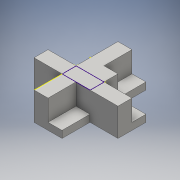
# Autodesk Inventor part: fourwayVer3
Saved by Autodesk Inventor 2016 (Build 200138000, 138)
## iProperties
Created: 2015-11-25
Part Number: fourwayVer3
Material: Generic
Document SubType Name: Modeling
Designer: hesaon
Density: 1 g/cm^3
Appearance: Default
Author: hesaon
Autodesk Inventor part; units mm, degrees
ref_plane "YZ Plane" through (0, 0, 0) normal (1, 0, 0) x (0, 1, 0)
ref_plane "XZ Plane" through (0, 0, 0) normal (0, 1, 0) x (-1, 0, 0)
ref_plane "XY Plane" through (0, 0, 0) normal (0, 0, 1) x (1, 0, 0)
sketch "Sketch1" plane through (0, 0, 0) normal (0, 0, 1) x (1, 0, 0)
  line L0 (0, 0) -> (12, 0)
  line L1 (12, 0) -> (12, 12)
  line L2 (12, 12) -> (0, 12)
  line L3 (0, 12) -> (0, 0)
  line L4 (12, 0) -> (0, 0)
  line L5 (0, 0) -> (0, -12)
  line L6 (0, -12) -> (12, -12)
  line L7 (12, -12) -> (12, 0)
  line L8 (12, 0) -> (24, 0)
  line L9 (24, 0) -> (24, -12)
  line L10 (24, -12) -> (12, -12)
  line L11 (12, -12) -> (12, 0)
  line L12 (0, -12) -> (-12, -12)
  line L13 (-12, -12) -> (-12, 0)
  line L14 (-12, 0) -> (0, 0)
  line L15 (0, 0) -> (0, -12)
  line L16 (0, -12) -> (12, -12)
  line L17 (12, -12) -> (12, -24)
  line L18 (12, -24) -> (0, -24)
  line L19 (0, -24) -> (0, -12)
  dimension "d0" = 12
  dimension "d1" = 12
  dimension "d2" = 12
  dimension "d3" = 12
  dimension "d4" = 12
  dimension "d5" = 12
  dimension "d6" = 12
  dimension "d7" = 12
  dimension "d8" = 12
  dimension "d9" = 12
  constraints: 40 end point, 10 parallel, 5 horizontal, 5 perpendicular
  measures "d0" distance of L2.end L1.end
  measures "d1" distance of L1.end L0.end
  measures "d2" distance of L6.end L5.end
  measures "d3" distance of L5.end L4.end
  measures "d4" distance of L9.end L10.end
  measures "d5" distance of L8.end L9.end
  measures "d6" distance of L13.end L14.end
  measures "d7" distance of L12.end L13.end
  measures "d8" distance of L17.end L18.end
  measures "d9" distance of L16.end L17.end
extrude "Extrusion1" add sketch "Sketch1" along normal blind 3
sketch "Sketch2" plane through (0, 0, 3) normal (0, 0, 1) x (1, 0, 0)
  line L0 (-12, 0) -> (-12, -12) projected
  line L1 (-12, -12) -> (-12, -6)
  line L2 (-12, -6) -> (0, -6)
  line L3 (-12, -12) -> (0, -12) projected
  line L4 (0, -6) -> (0, -12)
  line L5 (0, -12) -> (-12, -12)
  line L6 (12, -24) -> (12, -12) projected
  line L7 (12, -12) -> (12, -6)
  line L8 (12, -6) -> (24, -6)
  line L9 (24, -12) -> (24, 0) projected
  line L10 (12, -12) -> (24, -12) projected
  line L11 (24, -6) -> (24, -12)
  line L12 (24, -12) -> (12, -12)
  line L13 (0, 0) -> (0, -6)
  line L14 (12, 0) -> (12, 12) projected
  line L15 (0, 0) -> (12, 0)
  line L16 (12, 0) -> (12, -6)
  line L17 (12, -12) -> (0, -12)
  line L18 (0, 12) -> (0, 0) projected
  line L19 (0, 0) -> (0, 12)
  line L20 (0, 12) -> (6, 12)
  line L21 (12, 12) -> (0, 12) projected
  line L22 (6, 12) -> (6, 0)
  line L23 (6, 0) -> (0, 0)
  line L24 (0, -12) -> (0, -24) projected
  line L25 (0, -12) -> (0, -24)
  line L26 (0, -24) -> (6, -24)
  line L27 (0, -24) -> (12, -24) projected
  line L28 (6, -24) -> (6, -12)
  line L29 (6, -12) -> (0, -12)
  dimension "d12" = 6
  dimension "d13" = 12
  constraints: 40 end point, 6 collinear, 6 midpoint, 5 perpendicular, 2 horizontal, 1 vertical
  measures "d12" distance of L0.end L1.end
  measures "d13" distance of L8.end L7.end
extrude "Extrusion2" add sketch "Sketch2" along normal blind 9 contours L2 L4 L3 L0 | L13 L15 L16 L7 L17 L4 | L17 L28 L26 L24 | L18 L20 L22 L15 | L7 L8 L9 L10
sketch "Sketch3" plane through (0, 0, 12) normal (0, 0, 1) x (1, 0, 0)
  line L0 (0, -6) -> (12, -6)
  line L1 (12, -12) -> (6, -12) projected
  line L2 (12, -6) -> (12, -12)
  line L3 (0, -12) -> (0, -24) projected
  line L4 (12, -12) -> (0, -12)
  line L5 (0, -12) -> (0, -6)
  point P0 (0, 0)
  constraints: 8 end point, 3 perpendicular, 1 horizontal
body "Solid1"
